Joystick Keyboard Braces (Autodesk Fusion 360 design; units mm, degrees)
Autodesk Fusion 360 part; units mm, degrees
sketch "Sketch1" plane through (0, 0, 0) normal (0, 0, 1) x (1, 0, 0)
  line L0 (0, 0) -> (-60, 0)
  line L1 (-60, 0) -> (-60, 15)
  line L2 (-60, 15) -> (0, 15)
  line L3 (0, 15) -> (0, 0)
  line L4 (-60, 50) -> (0, 50)
  line L5 (0, 50) -> (0, 20)
  line L6 (0, 20) -> (-60, 20)
  line L7 (-60, 20) -> (-60, 50)
  dimension "d1" = 60
  dimension "d2" = 15
  dimension "d3" = 60
  dimension "d4" = 30
  constraint horizontal L0
  constraint vertical L1
  constraint horizontal L2
  constraint vertical L3
  constraint coincident L0.start L3.end
  constraint horizontal L6
  constraint vertical L7
  constraint horizontal L4
  constraint vertical L5
  measures "d1" distance of L0.start L0.end
  measures "d2" distance of L0.start L2.end
  measures "d3" distance of L5.end L6.end
  measures "d4" distance of L5.end L4.end
extrude "Extrude1" add sketch "Sketch1" along normal blind 2 makes body 1 at (-40, 30, 0) makes body 2 at (-20, 5, 0)
sketch "Sketch2" plane through (0, 0, 0) normal (0, 0, 1) x (1, 0, 0)
  line L0 (0, 76.0529) -> (11.4, 76.0529)
  line L1 (11.4, 76.0529) -> (11.4, 69.3529)
  line L2 (0, 69.3529) -> (0, 76.0529)
  line L3 (0, 62.6529) -> (0, 63.2769)
  line L4 (0, 62.6529) -> (11.4, 76.0529) construction
  line L5 (0, 76.0529) -> (11.4, 62.6529) construction
  line L6 (0.7, 69.3529) -> (0.7, 74.5246)
  line L7 (0.7, 74.5246) -> (10.6999, 74.4829)
  line L8 (10.6999, 74.4829) -> (10.6999, 69.3529)
  line L9 (10.7527, 64.2056) -> (0.7, 74.5246) construction
  line L10 (0.6714, 64.2531) -> (10.6999, 74.4829) construction
  arc A0 (4.2151, 67.8679) -> (4.3392, 67.7534) centre (5.7, 69.3529) ccw
  arc A1 (7.0608, 67.7534) -> (7.1849, 67.8679) centre (5.7, 69.3529) ccw
  arc A2 (7.8, 69.3529) -> (3.6, 69.3529) centre (5.7, 69.3529) ccw
  line L11 (11.4, 69.3529) -> (7.8, 69.3529)
  line L12 (3.6, 69.3529) -> (0, 69.3529)
  dimension "d7" = 11.4
  dimension "d8" = 13.4
  dimension "d9" = 10
  dimension "d11" = 4.2
  dimension "d20" = 0.7
  constraint horizontal L0
  constraint vertical L1
  constraint vertical L2
  constraint coincident L2 L3.end
  constraint parallel L6 L8
  constraint coincident A2.end L11
  constraint coincident L10 A0.start
  constraint coincident L4 A0.end
  constraint coincident L5 A1.start
  constraint concentric A0 A1
  constraint coincident L9 A1.end
  constraint concentric A1 A2
  constraint collinear L11 L12
  constraint coincident L12 L6.start
  constraint coincident L11 L8.end
  measures "d7" distance of L0.start L0.end
  measures "d8" distance of L0.start L3.start
  measures "d9" distance of L6.end L7.end
  measures "d11" diameter of A0
  measures "d20" distance of L2 L6
extrude "Extrude4" add sketch "Sketch2" along normal blind 10 separate body contours L0 L1 L2 L6 L7 L8 L11 L12 makes body 3
extrude "Extrude5" add sketch "Sketch2" along normal blind 7.5 contours L6 L7 L8 A2 L11 L12 bodies 3
